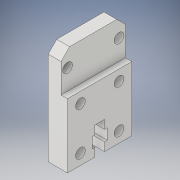
# Autodesk Inventor part: Spreader Frame
Saved by Autodesk Inventor 2018 (Build 220112000, 112)
## iProperties
Created: 2013-10-16
Part Number: Spreader Frame
Material: ASA Plastic
Document SubType Name: Modeling
Designer: Gabriel Smolnycki
Mass: 9.86644 g
Surface Area: 49.0685 cm^2
Volume: 9.22097 cm^3
Density: 1.07 g/cm^3
Appearance: Smooth - White ASA
Sending System: SolidWorks 2017
Last Author: Gabriel Smolnycki
Last Saved: 2017-09-14
Author: Gabriel Smolnycki
Autodesk Inventor part; units mm, degrees
ref_plane "XZ Plane" through (0, 0, 0) normal (0, 1, 0) x (-1, 0, 0)
ref_plane "XY Plane" through (0, 0, 0) normal (0, 0, 1) x (1, 0, 0)
ref_plane "Work Plane1" through (9, 0, 0) normal (1, 0, 0) x (0, 1, 0)
sketch "Sketch1" plane through (9, 0, 0) normal (1, 0, 0) x (0, 1, 0)
  line L0 (-30.5, 3.5) -> (-35.5, 3.5)
  line L1 (-30.5, 2.25) -> (-30.5, 3.5)
  line L2 (-26.5, 2.25) -> (-30.5, 2.25)
  line L3 (-26.5, -2.25) -> (-26.5, 2.25)
  line L4 (-30.5, -2.25) -> (-26.5, -2.25)
  line L5 (-30.5, -3.5) -> (-30.5, -2.25)
  line L6 (-35.5, 3.5) -> (-35.5, 2.25)
  line L7 (-35.5, -3.5) -> (-30.5, -3.5)
  line L8 (-35.5, -2.25) -> (-35.5, -3.5)
  line L9 (-39.5, -2.25) -> (-35.5, -2.25)
  line L10 (-39.5, -15) -> (-39.5, -2.25)
  line L11 (4, -15) -> (-39.5, -15)
  line L12 (8, -11) -> (4, -15)
  line L13 (8, 11) -> (8, -11)
  line L14 (4, 15) -> (8, 11)
  line L15 (-39.5, 15) -> (4, 15)
  line L16 (-39.5, 2.25) -> (-39.5, 15)
  line L17 (-35.5, 2.25) -> (-39.5, 2.25)
  constraints: 36 end point, 9 equal length, 8 horizontal, 8 vertical, 1 collinear, 1 perpendicular
extrude "Extrusion6" add sketch "Sketch1" against normal blind 9
sketch "Sketch2" plane through (0, 0, 0) normal (1, 0, 0) x (0, 1, 0)
  line L0 (-38, 11.0207) -> (-34.5, 13.0415)
  line L1 (-34.5, 4.9585) -> (-38, 6.9793)
  line L2 (-31, 6.9793) -> (-34.5, 4.9585)
  line L3 (-34.5, 13.0415) -> (-31, 11.0207)
  line L4 (-38, 6.9793) -> (-38, 11.0207)
  line L5 (-31, 11.0207) -> (-31, 6.9793)
  constraints: 12 end point, 5 equal length, 2 vertical
extrude "Extrusion5" cut sketch "Sketch2" along normal blind 5
sketch "Sketch3" plane through (0, 0, 0) normal (1, 0, 0) x (0, 1, 0)
  line L0 (-31, -11.0207) -> (-34.5, -13.0415)
  line L1 (-34.5, -4.9585) -> (-31, -6.9793)
  line L2 (-38, -11.0207) -> (-38, -6.9793)
  line L3 (-31, -6.9793) -> (-31, -11.0207)
  line L4 (-38, -6.9793) -> (-34.5, -4.9585)
  line L5 (-34.5, -13.0415) -> (-38, -11.0207)
  constraints: 12 end point, 5 equal length, 2 vertical
extrude "Extrusion4" cut sketch "Sketch3" along normal blind 5
sketch "Sketch4" plane through (0, 0, 0) normal (1, 0, 0) x (0, 1, 0)
  line L0 (-11, 11.0207) -> (-11, 6.9793)
  line L1 (-18, 11.0207) -> (-14.5, 13.0415)
  line L2 (-14.5, 4.9585) -> (-18, 6.9793)
  line L3 (-14.5, 13.0415) -> (-11, 11.0207)
  line L4 (-11, 6.9793) -> (-14.5, 4.9585)
  line L5 (-18, 6.9793) -> (-18, 11.0207)
  constraints: 12 end point, 5 equal length, 2 vertical
extrude "Extrusion3" cut sketch "Sketch4" along normal blind 5
sketch "Sketch5" plane through (0, 0, 0) normal (1, 0, 0) x (0, 1, 0)
  line L0 (-18, -11.0207) -> (-18, -6.9793)
  line L1 (-11, -11.0207) -> (-14.5, -13.0415)
  line L2 (-18, -6.9793) -> (-14.5, -4.9585)
  line L3 (-14.5, -13.0415) -> (-18, -11.0207)
  line L4 (-14.5, -4.9585) -> (-11, -6.9793)
  line L5 (-11, -6.9793) -> (-11, -11.0207)
  constraints: 12 end point, 5 equal length, 2 vertical
extrude "Extrusion2" cut sketch "Sketch5" along normal blind 5
sketch "Sketch6" plane through (9, 0, 0) normal (1, 0, 0) x (0, 1, 0)
  line L0 (4, 15) -> (-9.5, 15)
  line L1 (4, -15) -> (8, -11)
  line L2 (8, 11) -> (4, 15)
  line L3 (-9.5, -15) -> (4, -15)
  line L4 (-9.5, -15) -> (-9.5, 15)
  line L5 (8, -11) -> (8, 11)
  constraints: 12 end point, 2 equal length, 2 horizontal, 2 vertical, 1 perpendicular
extrude "Extrusion1" cut sketch "Sketch6" against normal blind 3
hole "Hole6" at (0, 0, -12) direction (1, 0, 0) diameter 4.5 depth 6
hole "Hole5" at (9, -14.5, -9) direction (-1, 0, 0) diameter 4.5 depth 4
hole "Hole4" at (9, -14.5, 9) direction (-1, 0, 0) diameter 4.5 depth 4
sketch "Sketch9" plane through (9, 0, 0) normal (1, 0, 0) x (0, 1, 0)
  point P0 (-14.5, 9)
hole "Hole3" at (9, -34.5, 9) direction (-1, 0, 0) diameter 4.5 depth 4
sketch "Sketch8" plane through (9, 0, 0) normal (1, 0, 0) x (0, 1, 0)
  point P0 (-14.5, -9)
hole "Hole2" at (9, -34.5, -9) direction (-1, 0, 0) diameter 4.5 depth 4
sketch "Sketch7" plane through (0, 0, 0) normal (1, 0, 0) x (0, 1, 0)
  point P0 (0, -12)
hole "Hole1" at (0, 0, 12) direction (1, 0, 0) diameter 4.5 depth 6
sketch "Sketch10" plane through (9, 0, 0) normal (1, 0, 0) x (0, 1, 0)
  point P0 (-34.5, 9)
sketch "Sketch11" plane through (9, 0, 0) normal (1, 0, 0) x (0, 1, 0)
  point P0 (-34.5, -9)
sketch "Sketch12" plane through (0, 0, 0) normal (1, 0, 0) x (0, 1, 0)
  point P0 (0, 12)
body "Solid3"
